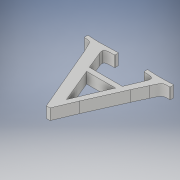
# Autodesk Inventor part: Letter_A
Saved by Autodesk Inventor 2019 (Build 230136000, 136)
## iProperties
Created: 2019-03-06
Part Number: Letter_A
Material: Generic
Document SubType Name: Modeling
Designer: jmc
Density: 1 g/cm^3
Appearance: Default
Author: jmc
## iProperties of the stored document Letter_A_3DPrint.ipt
Created: 2019-03-06
Part Number: Letter_A_3DPrint
Material: Generic
Document SubType Name: Modeling
Designer: jmc
Density: 1 g/cm^3
Appearance: Default
Author: jmc
Autodesk Inventor part; units mm, degrees
ref_plane "YZ Plane" through (0, 0, 0) normal (1, 0, 0) x (0, 1, 0)
ref_plane "XZ Plane" through (0, 0, 0) normal (0, 1, 0) x (-1, 0, 0)
ref_plane "XY Plane" through (0, 0, 0) normal (0, 0, 1) x (1, 0, 0)
sketch "Sketch1" plane through (0, 0, 0) normal (0, 1, 0) x (-1, 0, 0)
  line L0 (7.8064, 7.8064) -> (173.9884, 7.8064) construction
  line L1 (173.9884, 7.8064) -> (173.9884, -141.9122) construction
  line L2 (173.9884, -141.9122) -> (7.8064, -141.9122) construction
  line L3 (7.8064, -141.9122) -> (7.8064, 7.8064) construction
  line L4 (12.4499, -141.9122) -> (11.4649, -141.0679)
  line L5 (11.4649, -141.0679) -> (11.4649, -135.5801)
  line L6 (11.4649, -135.5801) -> (12.4499, -134.8765)
  spline S0 degree 2 poles (12.4499, -134.8765) (20.0484, -134.7358) (24.4105, -133.3287) (27.7877, -129.248) (32.994, -117.991) knots 0 0 0 1 2 3 3 3
  line L7 (32.994, -117.991) -> (43.9696, -94.2105)
  line L8 (43.9696, -94.2105) -> (72.3937, -30.0454)
  spline S1 degree 2 poles (72.3937, -30.0454) (80.4143, -11.0491) (88.2942, 7.8064) knots 0 0 0 1 1 1
  line L9 (88.2942, 7.8064) -> (95.0484, 7.8064)
  line L10 (95.0484, 7.8064) -> (139.6544, -96.884)
  line L11 (139.6544, -96.884) -> (145.5644, -110.9553)
  spline S2 degree 2 poles (145.5644, -110.9553) (148.2379, -116.8653) (154.9922, -130.7958) (157.525, -133.3287) (161.4649, -134.7358) (168.0785, -134.8765) knots 0 0 0 1 2 3 4 4 4
  line L12 (168.0785, -134.8765) -> (168.9227, -135.5801)
  line L13 (168.9227, -135.5801) -> (168.9227, -141.0679)
  line L14 (168.9227, -141.0679) -> (168.0785, -141.9122)
  spline S3 degree 2 poles (168.0785, -141.9122) (157.1028, -140.9272) (148.2379, -140.9272) knots 0 0 0 1 1 1
  spline S4 degree 2 poles (148.2379, -140.9272) (130.9302, -141.49) (113.6225, -141.9122) knots 0 0 0 1 1 1
  line L15 (113.6225, -141.9122) -> (112.7783, -141.0679)
  line L16 (112.7783, -141.0679) -> (112.7783, -135.5801)
  line L17 (112.7783, -135.5801) -> (113.6225, -134.8765)
  spline S5 degree 2 poles (113.6225, -134.8765) (125.3017, -134.5951) (131.071, -133.0472) (131.071, -130.233) knots 0 0 0 1 2 2 2
  spline S6 degree 2 poles (131.071, -130.233) (131.071, -127.9816) (129.6638, -124.1823) knots 0 0 0 1 1 1
  line L18 (129.6638, -124.1823) -> (116.8589, -92.3812)
  line L19 (116.8589, -92.3812) -> (56.3524, -92.3812)
  line L20 (56.3524, -92.3812) -> (45.0953, -119.1167)
  spline S7 degree 2 poles (45.0953, -119.1167) (41.9997, -126.293) (41.9997, -129.5294) knots 0 0 0 1 1 1
  spline S8 degree 2 poles (41.9997, -129.5294) (41.9997, -132.203) (47.6282, -134.7358) (59.0259, -134.8765) knots 0 0 0 1 2 2 2
  line L21 (59.0259, -134.8765) -> (60.0109, -135.5801)
  line L22 (60.0109, -135.5801) -> (60.0109, -141.0679)
  line L23 (60.0109, -141.0679) -> (59.1666, -141.9122)
  spline S9 degree 2 poles (59.1666, -141.9122) (45.6582, -141.0679) (35.5269, -141.0679) knots 0 0 0 1 1 1
  spline S10 degree 2 poles (35.5269, -141.0679) (24.1291, -141.0679) (12.4499, -141.9122) knots 0 0 0 1 1 1
  line L24 (60.0109, -83.3756) -> (112.7783, -83.3756)
  line L25 (112.7783, -83.3756) -> (86.6057, -20.4769)
  line L26 (86.6057, -20.4769) -> (60.0109, -83.3756)
  point P0 (0, 0)
  constraints: 2 other
extrude "Extrusion1" add sketch "Sketch1" along normal blind 20
body "Solid1"
